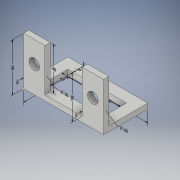
# Autodesk Inventor part: Actobotics Power Switch Mount
Saved by Autodesk Inventor 2018 (Build 220112000, 112)
## iProperties
Created: 2019-12-10
Part Number: Actobotics Power Switch Mount
Material: Generic
Document SubType Name: Modeling
Designer: AOFUser
Density: 1 g/cm^3
Appearance: Default
Author: AOFUser
Autodesk Inventor part; units mm, degrees
ref_plane "YZ Plane" through (0, 0, 0) normal (1, 0, 0) x (0, 1, 0)
ref_plane "XZ Plane" through (0, 0, 0) normal (0, 1, 0) x (-1, 0, 0)
ref_plane "XY Plane" through (0, 0, 0) normal (0, 0, 1) x (1, 0, 0)
sketch "Sketch1" plane through (0, 0, 0) normal (0, 1, 0) x (-1, 0, 0)
  point P0 (0, 0)
sketch "Sketch2" plane through (0, 0, 0) normal (0, 1, 0) x (-1, 0, 0)
  line L0 (0, 0) -> (-38.1, 0)
  line L1 (-38.1, 0) -> (-38.1, -21.082)
  line L2 (-38.1, -21.082) -> (0, -21.082)
  line L3 (0, -21.082) -> (0, 0)
  dimension "d0" = 38.1
  dimension "d1" = 21.082
  constraints: 8 end point, 2 parallel, 1 horizontal, 1 perpendicular
  measures "d0" distance of L2.end L1.end
  measures "d1" distance of L1.end L0.end
extrude "Extrusion1" add sketch "Sketch2" along normal blind 2.54
sketch "Sketch3" plane through (0, 2.54, 0) normal (0, 1, 0) x (1, 0, 0)
  line L0 (0, 0) -> (5.08, 0)
  line L1 (5.08, 0) -> (5.08, 5.08)
  line L2 (5.08, 5.08) -> (0, 5.08)
  line L3 (0, 5.08) -> (0, 0)
  line L4 (38.1, 0) -> (38.1, 21.082) projected
  line L5 (38.1, 21.082) -> (33.02, 21.082)
  line L6 (33.02, 21.082) -> (33.02, 16.002)
  line L7 (33.02, 16.002) -> (38.1, 16.002)
  line L8 (38.1, 16.002) -> (38.1, 21.082)
  line L9 (5.08, 5.08) -> (33.02, 5.08)
  line L10 (33.02, 5.08) -> (33.02, 16.002)
  line L11 (33.02, 16.002) -> (5.08, 16.002)
  line L12 (5.08, 16.002) -> (5.08, 5.08)
  dimension "d4" = 5.08
  dimension "d5" = 5.08
  dimension "d6" = 5.08
  dimension "d7" = 5.08
  constraints: 24 end point, 6 parallel, 3 horizontal, 3 perpendicular
  measures "d4" distance of L2.end L1.end
  measures "d5" distance of L1.end L0.end
  measures "d6" distance of L7.end L6.end
  measures "d7" distance of L6.end L5.end
extrude "Extrusion2" cut sketch "Sketch3" against normal blind 2.54 contours L12 L11 L10 L9
sketch "Sketch4" plane through (0, 2.54, 0) normal (0, 1, 0) x (1, 0, 0)
  line L0 (0, 0) -> (38.1, 0) projected
  line L1 (0, 0) -> (10.16, 0)
  line L2 (10.16, 0) -> (10.16, 2.54)
  line L3 (10.16, 2.54) -> (0, 2.54)
  line L4 (0, 2.54) -> (0, 0)
  line L5 (38.1, 0) -> (27.94, 0)
  line L6 (27.94, 0) -> (27.94, 2.54)
  line L7 (27.94, 2.54) -> (38.1, 2.54)
  line L8 (38.1, 2.54) -> (38.1, 0)
  dimension "d10" = 10.16
  dimension "d11" = 2.54
  dimension "d12" = 10.16
  dimension "d13" = 2.54
  constraints: 16 end point, 4 parallel, 2 horizontal, 2 perpendicular
  measures "d10" distance of L3.end L2.end
  measures "d11" distance of L2.end L1.end
  measures "d12" distance of L6.end L7.end
  measures "d13" distance of L5.end L6.end
extrude "Extrusion3" add sketch "Sketch4" along normal blind 20.32
sketch "Sketch5" plane through (10.16, 2.54, -2.54) normal (0, 0, -1) x (-1, 0, 0)
  line L0 (10.16, 20.32) -> (0, 20.32) projected
  line L1 (5.08, 20.32) -> (5.08, 10.16)
  point P0 (10.16, -2.54)
  dimension "d16" = 10.16
  constraints: 2 end point, 1 midpoint, 1 vertical
  measures "d16" distance of L1.start L1.end
hole "Hole1" at (5.08, 12.7, -2.54) direction (0, 0, 1) diameter 5.08 end through all
sketch "Sketch6" plane through (38.1, 2.54, -2.54) normal (0, 0, -1) x (-1, 0, 0)
  line L0 (10.16, 20.32) -> (0, 20.32) projected
  line L1 (5.08, 20.32) -> (5.08, 10.16)
  point P0 (38.1, -2.54)
  dimension "d24" = 10.16
  constraints: 2 end point, 1 midpoint, 1 vertical
  measures "d24" distance of L1.start L1.end
hole "Hole2" at (33.02, 12.7, -2.54) direction (0, 0, 1) diameter 5.08 end through all
body "Solid1"
